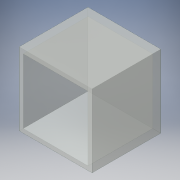
# Autodesk Inventor part: UQ-753-H100-40x40x100mm
Saved by Autodesk Inventor 2016 (Build 200138000, 138)
## iProperties
Created: 2016-07-06
Part Number: UQ-753-H100-40x40x100mm
Material: Glass
Document SubType Name: Modeling
Designer: voigt
Density: 2.18 g/cm^3
Appearance: Clear
Author: voigt
Autodesk Inventor part; units mm, degrees
ref_plane "YZ Plane" through (0, 0, 0) normal (1, 0, 0) x (0, 1, 0)
ref_plane "XZ Plane" through (0, 0, 0) normal (0, 1, 0) x (-1, 0, 0)
ref_plane "XY Plane" through (0, 0, 0) normal (0, 0, 1) x (1, 0, 0)
sketch "Sketch1" plane through (0, 0, 0) normal (0, 1, 0) x (-1, 0, 0)
  line L0 (0, -31.5) -> (0, 31.5) construction
  line L1 (-31.5, 0) -> (31.5, 0) construction
  line L2 (22.5, 22.5) -> (-22.5, 22.5)
  line L3 (-22.5, 22.5) -> (-22.5, -22.5)
  line L4 (-22.5, -22.5) -> (22.5, -22.5)
  line L5 (22.5, -22.5) -> (22.5, 22.5)
  line L6 (20, 20) -> (-20, 20)
  line L7 (-20, 20) -> (-20, -20)
  line L8 (-20, -20) -> (20, -20)
  line L9 (20, -20) -> (20, 20)
  point P0 (0, 0)
  dimension "d0" = 45
  dimension "d1" = 45
  dimension "d2" = 40
  dimension "d3" = 40
  constraints: 16 end point, 4 parallel, 2 horizontal, 2 perpendicular, 4 other
  measures "d0" distance of L3.end L4.end
  measures "d1" distance of L2.end L3.end
  measures "d2" distance of L8.end L7.end
  measures "d3" distance of L7.end L6.end
extrude "Extrusion1" add sketch "Sketch1" along normal blind 40
sketch "Sketch2" plane through (0, 40, 0) normal (0, 1, 0) x (1, 0, 0)
  line L0 (-22.5, 22.5) -> (-22.5, -22.5) projected
  line L1 (-22.5, -22.5) -> (22.5, -22.5) projected
  line L2 (22.5, -22.5) -> (22.5, 22.5) projected
  line L3 (22.5, 22.5) -> (-22.5, 22.5) projected
  point P0 (0, 0)
extrude "Extrusion2" add sketch "Sketch2" along normal blind 2.5
body "Solid1"
